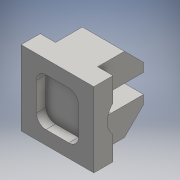
# Autodesk Inventor part: Cassetto
Saved by Autodesk Inventor 2016 (Build 200138000, 138)
## iProperties
Created: 2016-12-04
Part Number: Cassetto
Material: Generic
Document SubType Name: Modeling
Designer: Muhammad
Density: 1 g/cm^3
Appearance: Default
Author: Muhammad
Autodesk Inventor part; units mm, degrees
ref_plane "XZ Plane" through (0, 0, 0) normal (0, 1, 0) x (-1, 0, 0)
ref_plane "XY Plane" through (0, 0, 0) normal (0, 0, 1) x (1, 0, 0)
sketch "Sketch1" plane through (0, 0, 0) normal (0, 1, 0) x (-1, 0, 0)
  line L0 (9.5, 9.75) -> (-9.5, 9.75)
  line L1 (-9.5, 9.75) -> (-9.5, -9.75)
  line L2 (-9.5, -9.75) -> (9.5, -9.75)
  line L3 (9.5, -9.75) -> (9.5, 9.75)
  line L4 (9.5, 9.75) -> (-9.5, -9.75) construction
  line L5 (-9.5, 9.75) -> (9.5, -9.75) construction
  point P0 (0, 0)
  dimension "d0" = 19
  dimension "d1" = 19.5
  constraints: 12 end point, 2 midpoint, 2 parallel, 1 horizontal, 1 perpendicular
  measures "d0" distance of L2.end L1.end
  measures "d1" distance of L1.end L0.end
extrude "Extrusion1" add sketch "Sketch1" along normal blind 5
sketch "Sketch2" plane through (0, 0, 0) normal (0, -1, 0) x (1, 0, 0)
  line L0 (5.5, 6.2) -> (-5.5, 6.2)
  line L1 (-5.5, 6.2) -> (-5.5, -6.2)
  line L2 (-5.5, -6.2) -> (5.5, -6.2)
  line L3 (5.5, -6.2) -> (5.5, 6.2)
  line L4 (5.5, 6.2) -> (-5.5, -6.2) construction
  line L5 (-5.5, 6.2) -> (5.5, -6.2) construction
  point P0 (0, 0)
  dimension "d4" = 11
  dimension "d5" = 12.4
  constraints: 12 end point, 2 midpoint, 2 parallel, 1 horizontal, 1 perpendicular
  measures "d4" distance of L2.end L1.end
  measures "d5" distance of L1.end L0.end
extrude "Extrusion2" cut sketch "Sketch2" against normal blind 2.5
fillet "Fillet1" radius 2.5 4 edges at (-5.5, 1.25, 6.2) (5.5, 1.25, 6.2) (5.5, 1.25, -6.2) (-5.5, 1.25, -6.2)
sketch "Sketch3" plane through (0, 5, 0) normal (0, 1, 0) x (1, 0, 0)
  line L0 (9.5, 9.75) -> (-9.5, 9.75) projected
  line L1 (-5.5, -9.75) -> (5.5, -9.75)
  line L2 (5.5, -9.75) -> (5.5, 9.75)
  line L3 (5.5, 9.75) -> (-5.5, 9.75)
  line L4 (-5.5, 9.75) -> (-5.5, -9.75)
  line L5 (-5.5, -9.75) -> (5.5, 9.75) construction
  line L6 (5.5, -9.75) -> (-5.5, 9.75) construction
  point P0 (0, 0)
  dimension "d9" = 11
  constraints: 12 end point, 2 midpoint, 2 parallel, 1 horizontal, 1 perpendicular, 1 point on line
  measures "d9" distance of L3.end L2.end
extrude "Extrusion3" add sketch "Sketch3" along normal blind 12
chamfer "Chamfer1" distance 5 angle 45 2 edges at (0, 17, 9.75) (0, 17, -9.75)
sketch "Sketch4" plane through (5.5, 5, 9.75) normal (1, 0, 0) x (0, 0, -1)
  line L0 (12.25, 20.5) -> (7.25, 20.5)
  line L1 (7.25, 20.5) -> (7.25, 3.5)
  line L2 (7.25, 3.5) -> (12.25, 3.5)
  line L3 (12.25, 3.5) -> (12.25, 20.5)
  line L4 (14.5, 12) -> (5, 12) projected
  line L5 (12.25, 20.5) -> (7.25, 3.5) construction
  line L6 (7.25, 20.5) -> (12.25, 3.5) construction
  circle A0 centre (9.75, 3.5) radius 2.5
  point P0 (9.75, -5)
  point P1 (9.75, 12)
  dimension "d15" = 5
  dimension "d16" = 17
  constraints: 12 end point, 4 midpoint, 2 parallel, 1 horizontal, 1 horizontal alignment, 1 perpendicular, 2 other
  measures "d15" distance of L2.end L1.end
  measures "d16" distance of L1.end L0.end
extrude "Extrusion4" cut sketch "Sketch4" against normal through all
sketch "Sketch5" plane through (9.5, 0, 9.75) normal (1, 0, 0) x (0, 0, -1)
  arc A0 (7.25, 8.5) -> (12.25, 8.5) centre (9.75, 8.5) ccw projected
  circle A1 centre (9.75, 8.5) radius 5
  point P0 (9.75, 0)
  dimension "d19" = 10
  constraints: 1 centre point, 1 coincident
  measures "d19" diameter of A1
extrude "Extrusion5" cut sketch "Sketch5" against normal up to surface (4 mm away)
ref_plane "Work Plane1" through (0, 0, 0) normal (1, 0, 0) x (0, 1, 0)
mirror "Mirror1" about plane through (0, 0, 0) normal (1, 0, 0) of "Extrusion5"
body "Solid1"
